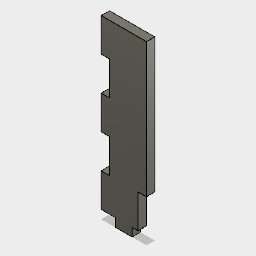
servo_guide1 v2 (Autodesk Fusion 360 design; units mm, degrees)
Autodesk Fusion 360 part; units mm, degrees
sketch "スケッチ1" plane through (0, 0, 0) normal (0, 0, 1) x (1, 0, 0)
  line L0 (19.2851, -21.7594) -> (19.2851, -31.7595)
  line L1 (19.2851, -31.7595) -> (16.7852, -31.7595)
  line L2 (16.7852, -21.7594) -> (19.2851, -21.7594)
  line L3 (16.7852, -41.7596) -> (19.2851, -41.7596)
  line L4 (16.7852, -31.7595) -> (16.7852, -41.7596)
  line L5 (16.7852, -11.7593) -> (16.7852, -21.7594)
  line L6 (21.0353, -61.7598) -> (21.0353, -64.2597)
  line L7 (19.2851, -41.7596) -> (19.2851, -51.7597)
  line L8 (30.2852, -11.7593) -> (16.7852, -11.7593)
  line L9 (21.0353, -64.2597) -> (26.0353, -64.2597)
  line L10 (27.7852, -51.7597) -> (30.2852, -51.7597)
  line L11 (26.0353, -61.7598) -> (27.7852, -61.7598)
  line L12 (16.7852, -51.7597) -> (16.7852, -61.7598)
  line L13 (16.7852, -61.7598) -> (21.0353, -61.7598)
  line L14 (19.2851, -51.7597) -> (16.7852, -51.7597)
  line L15 (26.0353, -64.2597) -> (26.0353, -61.7598)
  line L16 (27.7852, -61.7598) -> (27.7852, -51.7597)
  line L17 (30.2852, -51.7597) -> (30.2852, -11.7593)
extrude "押し出し1" add sketch "スケッチ1" along normal blind 2.5
